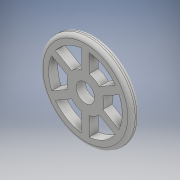
# Autodesk Inventor part: 보조바퀴
Saved by Autodesk Inventor 2018 (Build 220112000, 112)
## iProperties
Created: 2019-11-18
Part Number: 보조바퀴
Material: 일반
Document SubType Name: Modeling
Designer: LeeYounSeo
Density: 1 g/cm^3
Appearance: 기본값
Author: LeeYounSeo
Autodesk Inventor part; units mm, degrees
ref_plane "YZ Plane" through (0, 0, 0) normal (1, 0, 0) x (0, 1, 0)
ref_plane "XZ Plane" through (0, 0, 0) normal (0, 1, 0) x (-1, 0, 0)
ref_plane "XY Plane" through (0, 0, 0) normal (0, 0, 1) x (1, 0, 0)
sketch "스케치1" plane through (0, 0, 0) normal (0, 1, 0) x (-1, 0, 0)
  circle A0 centre (0, 0) radius 2.5
  circle A1 centre (0, 0) radius 12.5
  circle A2 centre (0, 0) radius 10
  circle A3 centre (0, 0) radius 5
  dimension "d0" = 5
  dimension "d1" = 25
  dimension "d2" = 20
  dimension "d3" = 10
  constraints: 4 centre point, 4 coincident
  measures "d0" diameter of A0
  measures "d1" diameter of A1
  measures "d2" diameter of A2
  measures "d3" diameter of A3
extrude "돌출1" add sketch "스케치1" along normal blind 2.5
sketch "스케치2" plane through (0, 2.5, 0) normal (0, 1, 0) x (1, 0, 0)
  line L0 (1, -11) -> (-1, -11)
  line L1 (-1, -11) -> (-1, 11)
  line L2 (-1, 11) -> (1, 11)
  line L3 (1, 11) -> (1, -11)
  circle A0 centre (0, 0) radius 10 projected
  dimension "d6" = 1
  dimension "d7" = 1
  dimension "d8" = 1
  dimension "d9" = 1
  constraints: 8 end point, 2 parallel, 1 horizontal, 1 perpendicular
  measures "d6" distance edge to line of A0 L2
  measures "d7" distance edge to line of A0 L0
  measures "d8" distance from line of point (0, 0) L1
  measures "d9" distance from line of point (0, 0) L3
extrude "돌출2" add sketch "스케치2" against normal blind 2.5 contours L0 L1 A0 L3 | A0 L1 L3 | A0 L1 L2 L3
pattern_circular "원형 패턴1" count 6 over 360 about axis through (0, 0, 0) along (0, 1, 0) of "돌출2"
sketch "스케치3" plane through (0, 2.5, 0) normal (0, 1, 0) x (1, 0, 0)
  line L0 (-2, 0) -> (-2.4843, 0.2796) projected
  circle A0 centre (0, 0) radius 2.5
  constraints: 1 coincident, 3 other
extrude "돌출3" cut sketch "스케치3" against normal blind 2.5
fillet "모깎기1" radius 1 2 edges at (12.5, 2.5, 0) (12.5, 0, 0)
